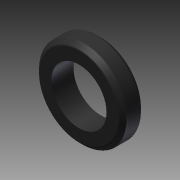
# Autodesk Inventor part: tire
Saved by Autodesk Inventor 2012 (Build 160160000, 160)
## iProperties
Created: 2011-10-06
Part Number: tire
Material: Default
Document SubType Name: Modeling
Designer: Antonella
Density: 1 g/cm^3
Author: Antonella
Autodesk Inventor part; units mm, degrees
ref_plane "YZ Plane" through (0, 0, 0) normal (1, 0, 0) x (0, 1, 0)
ref_plane "XZ Plane" through (0, 0, 0) normal (0, 1, 0) x (-1, 0, 0)
ref_plane "XY Plane" through (0, 0, 0) normal (0, 0, 1) x (1, 0, 0)
sketch "Sketch1" plane through (0, 0, 0) normal (0, 0, 1) x (1, 0, 0)
  circle A0 centre (0, 0) radius 203.2
  circle A1 centre (0, 0) radius 127
  dimension "d0" = 406.4
  dimension "d1" = 76.2
  constraints: 2 centre point, 1 coincident
  measures "d0" diameter of A0
  measures "d1" radial gap between concentric circles of A0 A1
extrude "Extrusion1" add sketch "Sketch1" along normal mid plane 101.6
chamfer "Chamfer1" distance 19.05 angle 45 2 edges at (-203.2, 0, 50.8) (-203.2, 0, -50.8)
fillet "Fillet2" radius 9.525 4 edges at (-203.2, 0, 31.75) (-184.15, 0, 50.8) (-203.2, 0, -31.75) (-184.15, 0, -50.8)
body "Solid1"
